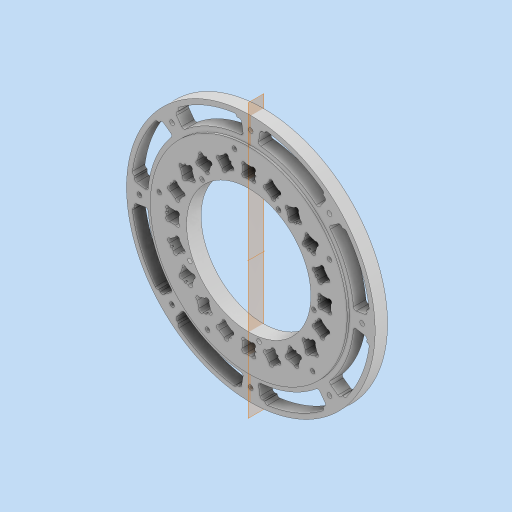
# Autodesk Inventor part: Ring_1
Saved by Autodesk Inventor 2024.2 (Build 282272000, 272)
## iProperties
Created: 2025-04-23
Part Number: Ring_1
Material: Generic
Document SubType Name: Modeling
Designer: 23661194
Density: 1 g/cm^3
Appearance: Default
Author: 23661194
Autodesk Inventor part; units mm, degrees
ref_plane "XZ Plane" through (0, 0, 0) normal (0, 1, 0) x (-1, 0, 0)
ref_plane "XY Plane" through (0, 0, 0) normal (0, 0, 1) x (1, 0, 0)
sketch "Shim Tray Slot" plane through (0, 0, 0) normal (0, 0, 1) x (1, 0, 0)
  line L0 (30.092, 109.0254) -> (29.9458, 108.3375)
  line L1 (33.5758, 105.3229) -> (31.6821, 97.1202)
  line L2 (-33.5758, 105.3229) -> (-31.6821, 97.1202)
  line L3 (-30.092, 109.0254) -> (-29.9458, 108.3375)
  arc A0 (-32.2001, 107.689) -> (-33.5758, 105.3229) centre (-31.6271, 105.7728) ccw
  arc A1 (29.1504, 95.657) -> (-29.1504, 95.657) centre (0, 0) ccw
  arc A2 (28.6337, 111.3782) -> (-28.6337, 111.3782) centre (0, 0) ccw
  arc A3 (-29.9458, 108.3375) -> (-32.2001, 107.689) centre (0, 0) ccw
  arc A4 (32.2001, 107.689) -> (29.9458, 108.3375) centre (0, 0) ccw
  arc A5 (-28.6337, 111.3782) -> (-30.092, 109.0254) centre (-28.1357, 109.4412) ccw
  arc A6 (-31.6821, 97.1202) -> (-29.1504, 95.657) centre (-29.7334, 97.5701) ccw
  arc A7 (29.1504, 95.657) -> (31.6821, 97.1202) centre (29.7309, 97.5743) ccw
  arc A8 (33.5758, 105.3229) -> (32.2001, 107.689) centre (31.6271, 105.7728) ccw
  arc A9 (30.092, 109.0254) -> (28.6337, 111.3782) centre (28.1357, 109.4412) ccw
  point P0 (0, 107.5)
  dimension "d173" = 22.5
sketch "Shim Tray Slot_1" plane through (0, 0, 0) normal (0, 0, 1) x (1, 0, 0)
  line L0 (30.092, 109.0254) -> (29.9458, 108.3375)
  line L1 (33.5758, 105.3229) -> (31.6829, 97.1237)
  line L2 (-33.5758, 105.3229) -> (-31.6821, 97.1202)
  line L3 (-30.092, 109.0254) -> (-29.9458, 108.3375)
  arc A0 (-32.2001, 107.689) -> (-33.5758, 105.3229) centre (-31.6271, 105.7728) ccw
  arc A1 (29.147, 95.658) -> (-29.1504, 95.657) centre (0, 0) ccw
  arc A2 (28.6337, 111.3782) -> (-28.6337, 111.3782) centre (0, 0) ccw
  arc A3 (-29.9458, 108.3375) -> (-32.2001, 107.689) centre (0, 0) ccw
  arc A4 (32.2001, 107.689) -> (29.9458, 108.3375) centre (0, 0) ccw
  arc A5 (-28.6337, 111.3782) -> (-30.092, 109.0254) centre (-28.1357, 109.4412) ccw
  arc A6 (-31.6821, 97.1202) -> (-29.1504, 95.657) centre (-29.7334, 97.5701) ccw
  arc A7 (29.147, 95.658) -> (31.6829, 97.1237) centre (29.7309, 97.5743) ccw
  arc A8 (33.5758, 105.3229) -> (32.2001, 107.689) centre (31.6271, 105.7728) ccw
  arc A9 (30.092, 109.0254) -> (28.6337, 111.3782) centre (28.1357, 109.4412) ccw
  line L4 (0, 0) -> (0, 107.5)
  arc A10 (33.9656, 105.2329) -> (32.3146, 108.0722) centre (31.6271, 105.7728) ccw
  line L5 (33.9656, 105.2329) -> (32.0726, 97.0337)
  arc A11 (29.0304, 95.2754) -> (32.0726, 97.0337) centre (29.7309, 97.5743) ccw
  arc A12 (29.0304, 95.2754) -> (-29.0338, 95.2743) centre (0, 0) ccw
  arc A13 (-32.0718, 97.0302) -> (-29.0338, 95.2743) centre (-29.7334, 97.5701) ccw
  line L6 (-32.0718, 97.0302) -> (-33.9656, 105.2329)
  arc A14 (-32.3146, 108.0722) -> (-33.9656, 105.2329) centre (-31.6271, 105.7728) ccw
  arc A15 (-30.4152, 108.6221) -> (-32.3146, 108.0722) centre (0, 0) ccw
  line L7 (-30.4152, 108.6221) -> (-30.4833, 108.9422)
  arc A16 (-28.7333, 111.7656) -> (-30.4833, 108.9422) centre (-28.1357, 109.4412) ccw
  arc A17 (28.7333, 111.7656) -> (-28.7333, 111.7656) centre (0, 0) ccw
  arc A18 (30.4833, 108.9422) -> (28.7333, 111.7656) centre (28.1357, 109.4412) ccw
  line L8 (30.4833, 108.9422) -> (30.4152, 108.6221)
  arc A19 (32.3146, 108.0722) -> (30.4152, 108.6221) centre (0, 0) ccw
  dimension "d182" = 0.4
  measures "d182" radial gap between concentric circles of A2 A17
sketch "Sketch1" plane through (0, 0, 0) normal (0, 0, 1) x (1, 0, 0)
  circle A0 centre (0, 0) radius 60
  circle A1 centre (0, 0) radius 120
  circle A2 centre (0, 0) radius 95
  dimension "d0" = 120
  dimension "d1" = 240
  dimension "d2" = 190
  constraints: 3 centre point, 3 coincident
  measures "d0" diameter of A0
  measures "d1" diameter of A1
  measures "d2" diameter of A2
extrude "Extrusion1" add sketch "Sketch1" along normal blind 12 contours A1 | A2
extrude "Extrusion2" add sketch "Sketch1" along normal blind 14 contours A2
sketch "Sketch2" plane through (0, 0, 14) normal (0, 0, 1) x (1, 0, 0)
  circle A0 centre (0, 0) radius 73.485
  line L0 (73.485, 0) -> (0, 0)
  line L1 (69.8884, 22.7081) -> (0, 0)
  line L2 (59.4506, 43.1934) -> (0, 0)
  line L3 (43.1934, 59.4506) -> (0, 0)
  line L4 (22.7081, 69.8884) -> (0, 0)
  line L5 (0, 73.485) -> (0, 0)
  line L6 (-22.7081, 69.8884) -> (0, 0)
  line L7 (-43.1934, 59.4506) -> (0, 0)
  line L8 (-59.4506, 43.1934) -> (0, 0)
  line L9 (-69.8884, 22.7081) -> (0, 0)
  line L10 (-73.485, 0) -> (0, 0)
  line L11 (-69.8884, -22.7081) -> (0, 0)
  line L12 (-59.4506, -43.1934) -> (0, 0)
  line L13 (-43.1934, -59.4506) -> (0, 0)
  line L14 (-22.7081, -69.8884) -> (0, 0)
  line L15 (0, -73.485) -> (0, 0)
  line L16 (22.7081, -69.8884) -> (0, 0)
  line L17 (43.1934, -59.4506) -> (0, 0)
  line L18 (59.4506, -43.1934) -> (0, 0)
  line L19 (69.8884, -22.7081) -> (0, 0)
  line L20 (-168, 0) -> (168, 0) projected
  line L21 (79.425, 5.94) -> (67.545, 5.94)
  line L22 (67.545, 5.94) -> (67.545, -5.94)
  line L23 (67.545, -5.94) -> (79.425, -5.94)
  line L24 (79.425, -5.94) -> (79.425, 5.94)
  line L25 (79.425, 5.94) -> (67.545, -5.94) construction
  line L26 (67.545, 5.94) -> (79.425, -5.94) construction
  circle A1 centre (73.485, 0) radius 2
  circle A2 centre (68.958, -4.527) radius 2.1
  circle A3 centre (78.012, -4.527) radius 2.1
  circle A4 centre (78.012, 4.527) radius 2.1
  circle A5 centre (68.958, 4.527) radius 2.1
  circle A6 centre (67.185, 0) radius 0.75
  line L27 (67.185, 0) -> (73.485, 0)
  line L28 (71.2025, 31.0051) -> (61.5914, 24.0222)
  line L29 (61.5914, 24.0222) -> (68.5743, 14.4111)
  line L30 (68.5743, 14.4111) -> (78.1854, 21.394)
  line L31 (78.1854, 21.394) -> (71.2025, 31.0051)
  line L32 (71.2025, 31.0051) -> (68.5743, 14.4111) construction
  line L33 (61.5914, 24.0222) -> (78.1854, 21.394) construction
  circle A7 centre (69.8884, 22.7081) radius 2
  circle A8 centre (68.8869, 16.3848) radius 2.1
  circle A9 centre (76.2117, 21.7066) radius 2.1
  circle A10 centre (70.8899, 29.0314) radius 2.1
  circle A11 centre (63.5651, 23.7096) radius 2.1
  circle A12 centre (64.7916, 19.0051) radius 0.75
  line L34 (64.7916, 19.0051) -> (69.8884, 22.7081)
  line L35 (55.6369, 50.6782) -> (51.9658, 39.3797)
  line L36 (51.9658, 39.3797) -> (63.2643, 35.7086)
  line L37 (63.2643, 35.7086) -> (66.9355, 47.0071)
  line L38 (66.9355, 47.0071) -> (55.6369, 50.6782)
  line L39 (55.6369, 50.6782) -> (63.2643, 35.7086) construction
  line L40 (51.9658, 39.3797) -> (66.9355, 47.0071) construction
  circle A13 centre (59.4506, 43.1934) radius 2
  circle A14 centre (62.3571, 37.489) radius 2.1
  circle A15 centre (65.155, 46.0999) radius 2.1
  circle A16 centre (56.5441, 48.8978) radius 2.1
  circle A17 centre (53.7463, 40.2869) radius 2.1
  circle A18 centre (57.5038, 37.2017) radius 0.75
  line L41 (57.5038, 37.2017) -> (59.4506, 43.1934)
  line L42 (35.7086, 63.2643) -> (39.3797, 51.9658)
  line L43 (39.3797, 51.9658) -> (50.6782, 55.6369)
  line L44 (50.6782, 55.6369) -> (47.0071, 66.9355)
  line L45 (47.0071, 66.9355) -> (35.7086, 63.2643)
  line L46 (35.7086, 63.2643) -> (50.6782, 55.6369) construction
  line L47 (39.3797, 51.9658) -> (47.0071, 66.9355) construction
  circle A19 centre (43.1934, 59.4506) radius 2
  circle A20 centre (48.8978, 56.5441) radius 2.1
  circle A21 centre (46.0999, 65.155) radius 2.1
  circle A22 centre (37.489, 62.3571) radius 2.1
  circle A23 centre (40.2869, 53.7463) radius 2.1
  circle A24 centre (45.1402, 53.459) radius 0.75
  line L48 (45.1402, 53.459) -> (43.1934, 59.4506)
  line L49 (14.4111, 68.5743) -> (24.0222, 61.5914)
  line L50 (24.0222, 61.5914) -> (31.0051, 71.2025)
  line L51 (31.0051, 71.2025) -> (21.394, 78.1854)
  line L52 (21.394, 78.1854) -> (14.4111, 68.5743)
  line L53 (14.4111, 68.5743) -> (31.0051, 71.2025) construction
  line L54 (24.0222, 61.5914) -> (21.394, 78.1854) construction
  circle A25 centre (22.7081, 69.8884) radius 2
  circle A26 centre (29.0314, 70.8899) radius 2.1
  circle A27 centre (21.7066, 76.2117) radius 2.1
  circle A28 centre (16.3848, 68.8869) radius 2.1
  circle A29 centre (23.7096, 63.5651) radius 2.1
  circle A30 centre (27.8049, 66.1853) radius 0.75
  line L55 (27.8049, 66.1853) -> (22.7081, 69.8884)
  line L56 (-5.94, 67.545) -> (5.94, 67.545)
  line L57 (5.94, 67.545) -> (5.94, 79.425)
  line L58 (5.94, 79.425) -> (-5.94, 79.425)
  line L59 (-5.94, 79.425) -> (-5.94, 67.545)
  line L60 (-5.94, 67.545) -> (5.94, 79.425) construction
  line L61 (5.94, 67.545) -> (-5.94, 79.425) construction
  circle A31 centre (0, 73.485) radius 2
  circle A32 centre (4.527, 78.012) radius 2.1
  circle A33 centre (-4.527, 78.012) radius 2.1
  circle A34 centre (-4.527, 68.958) radius 2.1
  circle A35 centre (4.527, 68.958) radius 2.1
  circle A36 centre (6.3, 73.485) radius 0.75
  line L62 (6.3, 73.485) -> (0, 73.485)
  line L63 (-24.0222, 61.5914) -> (-14.4111, 68.5743)
  line L64 (-14.4111, 68.5743) -> (-21.394, 78.1854)
  line L65 (-21.394, 78.1854) -> (-31.0051, 71.2025)
  line L66 (-31.0051, 71.2025) -> (-24.0222, 61.5914)
  line L67 (-24.0222, 61.5914) -> (-21.394, 78.1854) construction
  line L68 (-14.4111, 68.5743) -> (-31.0051, 71.2025) construction
  circle A37 centre (-22.7081, 69.8884) radius 2
  circle A38 centre (-21.7066, 76.2117) radius 2.1
  circle A39 centre (-29.0314, 70.8899) radius 2.1
  circle A40 centre (-23.7096, 63.5651) radius 2.1
  circle A41 centre (-16.3848, 68.8869) radius 2.1
  circle A42 centre (-17.6113, 73.5914) radius 0.75
  line L69 (-17.6113, 73.5914) -> (-22.7081, 69.8884)
  line L70 (-39.3797, 51.9658) -> (-35.7086, 63.2643)
  line L71 (-35.7086, 63.2643) -> (-47.0071, 66.9355)
  line L72 (-47.0071, 66.9355) -> (-50.6782, 55.6369)
  line L73 (-50.6782, 55.6369) -> (-39.3797, 51.9658)
  line L74 (-39.3797, 51.9658) -> (-47.0071, 66.9355) construction
  line L75 (-35.7086, 63.2643) -> (-50.6782, 55.6369) construction
  circle A43 centre (-43.1934, 59.4506) radius 2
  circle A44 centre (-46.0999, 65.155) radius 2.1
  circle A45 centre (-48.8978, 56.5441) radius 2.1
  circle A46 centre (-40.2869, 53.7463) radius 2.1
  circle A47 centre (-37.489, 62.3571) radius 2.1
  circle A48 centre (-41.2466, 65.4423) radius 0.75
  line L76 (-41.2466, 65.4423) -> (-43.1934, 59.4506)
  line L77 (-51.9658, 39.3797) -> (-55.6369, 50.6782)
  line L78 (-55.6369, 50.6782) -> (-66.9355, 47.0071)
  line L79 (-66.9355, 47.0071) -> (-63.2643, 35.7086)
  line L80 (-63.2643, 35.7086) -> (-51.9658, 39.3797)
  line L81 (-51.9658, 39.3797) -> (-66.9355, 47.0071) construction
  line L82 (-55.6369, 50.6782) -> (-63.2643, 35.7086) construction
  circle A49 centre (-59.4506, 43.1934) radius 2
  circle A50 centre (-65.155, 46.0999) radius 2.1
  circle A51 centre (-62.3571, 37.489) radius 2.1
  circle A52 centre (-53.7463, 40.2869) radius 2.1
  circle A53 centre (-56.5441, 48.8978) radius 2.1
  circle A54 centre (-61.3974, 49.1851) radius 0.75
  line L83 (-61.3974, 49.1851) -> (-59.4506, 43.1934)
  line L84 (-61.5914, 24.0222) -> (-71.2025, 31.0051)
  line L85 (-71.2025, 31.0051) -> (-78.1854, 21.394)
  line L86 (-78.1854, 21.394) -> (-68.5743, 14.4111)
  line L87 (-68.5743, 14.4111) -> (-61.5914, 24.0222)
  line L88 (-61.5914, 24.0222) -> (-78.1854, 21.394) construction
  line L89 (-71.2025, 31.0051) -> (-68.5743, 14.4111) construction
  circle A55 centre (-69.8884, 22.7081) radius 2
  circle A56 centre (-76.2117, 21.7066) radius 2.1
  circle A57 centre (-68.8869, 16.3848) radius 2.1
  circle A58 centre (-63.5651, 23.7096) radius 2.1
  circle A59 centre (-70.8899, 29.0314) radius 2.1
  circle A60 centre (-74.9852, 26.4112) radius 0.75
  line L90 (-74.9852, 26.4112) -> (-69.8884, 22.7081)
  line L91 (-67.545, 5.94) -> (-79.425, 5.94)
  line L92 (-79.425, 5.94) -> (-79.425, -5.94)
  line L93 (-79.425, -5.94) -> (-67.545, -5.94)
  line L94 (-67.545, -5.94) -> (-67.545, 5.94)
  line L95 (-67.545, 5.94) -> (-79.425, -5.94) construction
  line L96 (-79.425, 5.94) -> (-67.545, -5.94) construction
  circle A61 centre (-73.485, 0) radius 2
  circle A62 centre (-78.012, -4.527) radius 2.1
  circle A63 centre (-68.958, -4.527) radius 2.1
  circle A64 centre (-68.958, 4.527) radius 2.1
  circle A65 centre (-78.012, 4.527) radius 2.1
  circle A66 centre (-79.785, 0) radius 0.75
  line L97 (-79.785, 0) -> (-73.485, 0)
  line L98 (-68.5743, -14.4111) -> (-78.1854, -21.394)
  line L99 (-78.1854, -21.394) -> (-71.2025, -31.0051)
  line L100 (-71.2025, -31.0051) -> (-61.5914, -24.0222)
  line L101 (-61.5914, -24.0222) -> (-68.5743, -14.4111)
  line L102 (-68.5743, -14.4111) -> (-71.2025, -31.0051) construction
  line L103 (-78.1854, -21.394) -> (-61.5914, -24.0222) construction
  circle A67 centre (-69.8884, -22.7081) radius 2
  circle A68 centre (-70.8899, -29.0314) radius 2.1
  circle A69 centre (-63.5651, -23.7096) radius 2.1
  circle A70 centre (-68.8869, -16.3848) radius 2.1
  circle A71 centre (-76.2117, -21.7066) radius 2.1
  circle A72 centre (-74.9852, -26.4112) radius 0.75
  line L104 (-74.9852, -26.4112) -> (-69.8884, -22.7081)
  line L105 (-63.2643, -35.7086) -> (-66.9355, -47.0071)
  line L106 (-66.9355, -47.0071) -> (-55.6369, -50.6782)
  line L107 (-55.6369, -50.6782) -> (-51.9658, -39.3797)
  line L108 (-51.9658, -39.3797) -> (-63.2643, -35.7086)
  line L109 (-63.2643, -35.7086) -> (-55.6369, -50.6782) construction
  line L110 (-66.9355, -47.0071) -> (-51.9658, -39.3797) construction
  circle A73 centre (-59.4506, -43.1934) radius 2
  circle A74 centre (-56.5441, -48.8978) radius 2.1
  circle A75 centre (-53.7463, -40.2869) radius 2.1
  circle A76 centre (-62.3571, -37.489) radius 2.1
  circle A77 centre (-65.155, -46.0999) radius 2.1
  circle A78 centre (-61.3974, -49.1851) radius 0.75
  line L111 (-61.3974, -49.1851) -> (-59.4506, -43.1934)
  line L112 (-50.6782, -55.6369) -> (-47.0071, -66.9355)
  line L113 (-47.0071, -66.9355) -> (-35.7086, -63.2643)
  line L114 (-35.7086, -63.2643) -> (-39.3797, -51.9658)
  line L115 (-39.3797, -51.9658) -> (-50.6782, -55.6369)
  line L116 (-50.6782, -55.6369) -> (-35.7086, -63.2643) construction
  line L117 (-47.0071, -66.9355) -> (-39.3797, -51.9658) construction
  circle A79 centre (-43.1934, -59.4506) radius 2
  circle A80 centre (-37.489, -62.3571) radius 2.1
  circle A81 centre (-40.2869, -53.7463) radius 2.1
  circle A82 centre (-48.8978, -56.5441) radius 2.1
  circle A83 centre (-46.0999, -65.155) radius 2.1
  circle A84 centre (-41.2466, -65.4423) radius 0.75
  line L118 (-41.2466, -65.4423) -> (-43.1934, -59.4506)
  line L119 (-31.0051, -71.2025) -> (-21.394, -78.1854)
  line L120 (-21.394, -78.1854) -> (-14.4111, -68.5743)
  line L121 (-14.4111, -68.5743) -> (-24.0222, -61.5914)
  line L122 (-24.0222, -61.5914) -> (-31.0051, -71.2025)
  line L123 (-31.0051, -71.2025) -> (-14.4111, -68.5743) construction
  line L124 (-21.394, -78.1854) -> (-24.0222, -61.5914) construction
  circle A85 centre (-22.7081, -69.8884) radius 2
  circle A86 centre (-16.3848, -68.8869) radius 2.1
  circle A87 centre (-23.7096, -63.5651) radius 2.1
  circle A88 centre (-29.0314, -70.8899) radius 2.1
  circle A89 centre (-21.7066, -76.2117) radius 2.1
  circle A90 centre (-17.6113, -73.5914) radius 0.75
  line L125 (-17.6113, -73.5914) -> (-22.7081, -69.8884)
  line L126 (-5.94, -79.425) -> (5.94, -79.425)
  line L127 (5.94, -79.425) -> (5.94, -67.545)
  line L128 (5.94, -67.545) -> (-5.94, -67.545)
  line L129 (-5.94, -67.545) -> (-5.94, -79.425)
  line L130 (-5.94, -79.425) -> (5.94, -67.545) construction
  line L131 (5.94, -79.425) -> (-5.94, -67.545) construction
  circle A91 centre (0, -73.485) radius 2
  circle A92 centre (4.527, -68.958) radius 2.1
  circle A93 centre (-4.527, -68.958) radius 2.1
  circle A94 centre (-4.527, -78.012) radius 2.1
  circle A95 centre (4.527, -78.012) radius 2.1
  circle A96 centre (6.3, -73.485) radius 0.75
  line L132 (6.3, -73.485) -> (0, -73.485)
  line L133 (21.394, -78.1854) -> (31.0051, -71.2025)
  line L134 (31.0051, -71.2025) -> (24.0222, -61.5914)
  line L135 (24.0222, -61.5914) -> (14.4111, -68.5743)
  line L136 (14.4111, -68.5743) -> (21.394, -78.1854)
  line L137 (21.394, -78.1854) -> (24.0222, -61.5914) construction
  line L138 (31.0051, -71.2025) -> (14.4111, -68.5743) construction
  circle A97 centre (22.7081, -69.8884) radius 2
  circle A98 centre (23.7096, -63.5651) radius 2.1
  circle A99 centre (16.3848, -68.8869) radius 2.1
  circle A100 centre (21.7066, -76.2117) radius 2.1
  circle A101 centre (29.0314, -70.8899) radius 2.1
  circle A102 centre (27.8049, -66.1853) radius 0.75
  line L139 (27.8049, -66.1853) -> (22.7081, -69.8884)
  line L140 (78.1854, -21.394) -> (68.5743, -14.4111)
  line L141 (68.5743, -14.4111) -> (61.5914, -24.0222)
  line L142 (61.5914, -24.0222) -> (71.2025, -31.0051)
  line L143 (71.2025, -31.0051) -> (78.1854, -21.394)
  line L144 (78.1854, -21.394) -> (61.5914, -24.0222) construction
  line L145 (68.5743, -14.4111) -> (71.2025, -31.0051) construction
  circle A103 centre (69.8884, -22.7081) radius 2
  circle A104 centre (63.5651, -23.7096) radius 2.1
  circle A105 centre (70.8899, -29.0314) radius 2.1
  circle A106 centre (76.2117, -21.7066) radius 2.1
  circle A107 centre (68.8869, -16.3848) radius 2.1
  circle A108 centre (64.7916, -19.0051) radius 0.75
  line L146 (64.7916, -19.0051) -> (69.8884, -22.7081)
  line L147 (47.0071, -66.9355) -> (50.6782, -55.6369)
  line L148 (50.6782, -55.6369) -> (39.3797, -51.9658)
  line L149 (39.3797, -51.9658) -> (35.7086, -63.2643)
  line L150 (35.7086, -63.2643) -> (47.0071, -66.9355)
  line L151 (47.0071, -66.9355) -> (39.3797, -51.9658) construction
  line L152 (50.6782, -55.6369) -> (35.7086, -63.2643) construction
  circle A109 centre (43.1934, -59.4506) radius 2
  circle A110 centre (40.2869, -53.7463) radius 2.1
  circle A111 centre (37.489, -62.3571) radius 2.1
  circle A112 centre (46.0999, -65.155) radius 2.1
  circle A113 centre (48.8978, -56.5441) radius 2.1
  circle A114 centre (45.1402, -53.459) radius 0.75
  line L153 (45.1402, -53.459) -> (43.1934, -59.4506)
  line L154 (66.9355, -47.0071) -> (63.2643, -35.7086)
  line L155 (63.2643, -35.7086) -> (51.9658, -39.3797)
  line L156 (51.9658, -39.3797) -> (55.6369, -50.6782)
  line L157 (55.6369, -50.6782) -> (66.9355, -47.0071)
  line L158 (66.9355, -47.0071) -> (51.9658, -39.3797) construction
  line L159 (63.2643, -35.7086) -> (55.6369, -50.6782) construction
  circle A115 centre (59.4506, -43.1934) radius 2
  circle A116 centre (53.7463, -40.2869) radius 2.1
  circle A117 centre (56.5441, -48.8978) radius 2.1
  circle A118 centre (65.155, -46.0999) radius 2.1
  circle A119 centre (62.3571, -37.489) radius 2.1
  circle A120 centre (57.5038, -37.2017) radius 0.75
  line L160 (57.5038, -37.2017) -> (59.4506, -43.1934)
  point P0 (68.8025, -29.2614)
  point P1 (72.9462, -28.6052)
  point P2 (76.4417, -23.794)
  point P3 (75.7854, -19.6503)
  point P4 (70.9742, -16.1548)
  point P5 (66.8306, -16.8111)
  point P6 (63.3351, -21.6223)
  point P7 (63.9913, -25.7659)
  point P8 (52.8825, -42.201)
  point P9 (54.7202, -47.8569)
  point P10 (58.4582, -49.7615)
  point P11 (64.1141, -47.9238)
  point P12 (66.0187, -44.1858)
  point P13 (64.181, -38.5299)
  point P14 (60.443, -36.6253)
  point P15 (54.7871, -38.463)
  point P16 (36.6253, -60.443)
  point P17 (38.5299, -64.181)
  point P18 (44.1858, -66.0187)
  point P19 (47.9238, -64.1141)
  point P20 (49.7615, -58.4582)
  point P21 (47.8569, -54.7202)
  point P22 (42.201, -52.8825)
  point P23 (38.463, -54.7871)
  point P24 (19.6503, -75.7854)
  point P25 (23.794, -76.4417)
  point P26 (28.6052, -72.9462)
  point P27 (29.2614, -68.8025)
  point P28 (25.7659, -63.9913)
  point P29 (21.6223, -63.3351)
  point P30 (16.8111, -66.8306)
  point P31 (16.1548, -70.9742)
  point P32 (5.94, -70.5115)
  point P33 (2.9735, -67.545)
  point P34 (-2.9735, -67.545)
  point P35 (-5.94, -70.5115)
  point P36 (-5.94, -76.4585)
  point P37 (-2.9735, -79.425)
  point P38 (2.9735, -79.425)
  point P39 (5.94, -76.4585)
  point P40 (-21.6223, -63.3351)
  point P41 (-25.7659, -63.9913)
  point P42 (-29.2614, -68.8025)
  point P43 (-28.6052, -72.9462)
  point P44 (-23.794, -76.4417)
  point P45 (-19.6503, -75.7854)
  point P46 (-16.1548, -70.9742)
  point P47 (-16.8111, -66.8306)
  point P48 (-49.7615, -58.4582)
  point P49 (-47.9238, -64.1141)
  point P50 (-44.1858, -66.0187)
  point P51 (-38.5299, -64.181)
  point P52 (-36.6253, -60.443)
  point P53 (-38.463, -54.7871)
  point P54 (-42.201, -52.8825)
  point P55 (-47.8569, -54.7202)
  point P56 (-54.7202, -47.8569)
  point P57 (-52.8825, -42.201)
  point P58 (-54.7871, -38.463)
  point P59 (-60.443, -36.6253)
  point P60 (-64.181, -38.5299)
  point P61 (-66.0187, -44.1858)
  point P62 (-64.1141, -47.9238)
  point P63 (-58.4582, -49.7615)
  point P64 (-66.8306, -16.8111)
  point P65 (-70.9742, -16.1548)
  point P66 (-75.7854, -19.6503)
  point P67 (-76.4417, -23.794)
  point P68 (-72.9462, -28.6052)
  point P69 (-68.8025, -29.2614)
  point P70 (-63.9913, -25.7659)
  point P71 (-63.3351, -21.6223)
  point P72 (-67.545, 2.9735)
  point P73 (-70.5115, 5.94)
  point P74 (-76.4585, 5.94)
  point P75 (-79.425, 2.9735)
  point P76 (-79.425, -2.9735)
  point P77 (-76.4585, -5.94)
  point P78 (-70.5115, -5.94)
  point P79 (-67.545, -2.9735)
  point P80 (-63.3351, 21.6223)
  point P81 (-63.9913, 25.7659)
  point P82 (-68.8025, 29.2614)
  point P83 (-72.9462, 28.6052)
  point P84 (-76.4417, 23.794)
  point P85 (-75.7854, 19.6503)
  point P86 (-70.9742, 16.1548)
  point P87 (-66.8306, 16.8111)
  point P88 (-54.7871, 38.463)
  point P89 (-52.8825, 42.201)
  point P90 (-54.7202, 47.8569)
  point P91 (-58.4582, 49.7615)
  point P92 (-64.1141, 47.9238)
  point P93 (-66.0187, 44.1858)
  point P94 (-64.181, 38.5299)
  point P95 (-60.443, 36.6253)
  point P96 (-42.201, 52.8825)
  point P97 (-38.463, 54.7871)
  point P98 (-36.6253, 60.443)
  point P99 (-38.5299, 64.181)
  point P100 (-44.1858, 66.0187)
  point P101 (-47.9238, 64.1141)
  point P102 (-49.7615, 58.4582)
  point P103 (-47.8569, 54.7202)
  point P104 (-16.8111, 66.8306)
  point P105 (-16.1548, 70.9742)
  point P106 (-19.6503, 75.7854)
  point P107 (-23.794, 76.4417)
  point P108 (-28.6052, 72.9462)
  point P109 (-29.2614, 68.8025)
  point P110 (-25.7659, 63.9913)
  point P111 (-21.6223, 63.3351)
  point P112 (-5.94, 70.5115)
  point P113 (-2.9735, 67.545)
  point P114 (2.9735, 67.545)
  point P115 (5.94, 70.5115)
  point P116 (5.94, 76.4585)
  point P117 (2.9735, 79.425)
  point P118 (-2.9735, 79.425)
  point P119 (-5.94, 76.4585)
  point P120 (16.1548, 70.9742)
  point P121 (16.8111, 66.8306)
  point P122 (21.6223, 63.3351)
  point P123 (25.7659, 63.9913)
  point P124 (29.2614, 68.8025)
  point P125 (28.6052, 72.9462)
  point P126 (23.794, 76.4417)
  point P127 (19.6503, 75.7854)
  point P128 (36.6253, 60.443)
  point P129 (38.463, 54.7871)
  point P130 (42.201, 52.8825)
  point P131 (47.8569, 54.7202)
  point P132 (49.7615, 58.4582)
  point P133 (47.9238, 64.1141)
  point P134 (44.1858, 66.0187)
  point P135 (38.5299, 64.181)
  point P136 (64.181, 38.5299)
  point P137 (66.0187, 44.1858)
  point P138 (64.1141, 47.9238)
  point P139 (58.4582, 49.7615)
  point P140 (54.7202, 47.8569)
  point P141 (52.8825, 42.201)
  point P142 (54.7871, 38.463)
  point P143 (60.443, 36.6253)
  point P144 (63.9913, 25.7659)
  point P145 (63.3351, 21.6223)
  point P146 (66.8306, 16.8111)
  point P147 (70.9742, 16.1548)
  point P148 (75.7854, 19.6503)
  point P149 (76.4417, 23.794)
  point P150 (72.9462, 28.6052)
  point P151 (68.8025, 29.2614)
  point P152 (70.5115, 5.94)
  point P153 (67.545, 2.9735)
  point P154 (67.545, -2.9735)
  point P155 (70.5115, -5.94)
  point P156 (76.4585, -5.94)
  point P157 (79.425, -2.9735)
  point P158 (79.425, 2.9735)
  point P159 (76.4585, 5.94)
  dimension "d7" = 146.97
  dimension "d123" = -36
  dimension "d124" = -72
  dimension "d125" = -108
  dimension "d126" = -144
  dimension "d127" = -180
  dimension "d128" = -216
  dimension "d129" = -252
  dimension "d130" = -288
  dimension "d131" = -324
  dimension "d132" = 0
  dimension "d133" = -36
  dimension "d134" = -72
  dimension "d135" = -108
  dimension "d136" = -144
  dimension "d137" = 180
  dimension "d138" = -216
  dimension "d139" = -252
  dimension "d140" = -288
  dimension "d141" = -324
  dimension "d120" = 360
  dimension "d122" = 0
  constraints: 40 end point, 2 horizontal, 1 coincident, 1 horizontal alignment, 84 other
  measures "d122" vertical extent of L0
extrude "Extrusion3" cut sketch "Sketch2" against normal blind 12 contours L0 A1 A0 | L20 A1 A0 | A0 A1 L0 | A0 A1 L20 | A1 L0 A6 L22 A5 L21 A0 | A0 L21 A4 L24 L20 A1 | A1 L20 L24 A3 L23 A0 | A0 L23 A2 L22 A6 L0 A1 | A6 L22 L0 | L0 L22 A6 | L30 A8 L29 A12 L34 A7 A0 | A0 A7 L28 A10 L31 A9 L30 | A4 L24 L21 | L21 L24 A4 | A5 L22 L21 | L21 L22 A5 | L140 A106 L143 A105 L142 A0 A103 | A0 A103 L146 A108 L141 A107 L140 | A2 L22 L23 | L23 L22 A2 | A3 L24 L23 | L23 L24 A3 | A7 L34 A0 | A0 A7 | A8 L29 L30 | L30 L29 A8 | A9 L31 L30 | L30 L31 A9 | A103 A0 | A0 L146 A103 | A106 L143 L140 | L140 L143 A106 | A107 L141 L140 | L140 L141 A107 | L1 A7 A0 | L34 A7 L1 | L34 A12 L29 L1 A7 | A0 A103 L19 | L19 A103 L146 | A103 L19 L141 A108 L146 | A7 L1 L29 A11 L28 A0 | L34 L29 A12 | A12 L29 L34 | A10 L28 L31 | L31 L28 A10 | A0 L142 A104 L141 L19 A103 | L146 L141 A108 | A108 L141 L146 | A105 L142 L143 | L143 L142 A105 | A17 L35 L36 L2 | L2 L36 A17 | A23 L42 L3 | L3 L42 L43 A23 | L49 A28 L52 A0 A25 L4 | L4 A25 L55 A30 L50 A29 L49 | L56 A34 L59 A0 A31 L5 | L5 A31 A0 A36 L57 A35 L56 | L63 A40 L66 A0 A37 L6 | L6 A37 A0 L64 A41 L63 | A46 L73 L70 L7 | L7 L70 A46 | A52 L80 L8 | L8 L80 L77 A52 | L87 A57 L86 A0 A55 L9 | L9 A55 A0 L84 A58 L87 | L94 A63 L93 A0 A61 L10 | L10 A61 A0 L91 A64 L94 | L101 A69 L100 A0 A67 L11 | L11 A67 A0 L98 A70 L101 | A75 L107 L108 L12 | L12 L108 A75 | A81 L114 L13 | L13 L114 L115 A81 | L121 A86 L120 A0 A85 L14 | L14 A85 A0 L122 A87 L121 | L128 A92 L127 A96 A0 A91 L15 | L15 A91 A0 L129 A93 L128 | L135 A98 L134 A102 L139 A97 L16 | L16 A97 A0 L136 A99 L135 | A110 L148 L149 L17 | L17 L149 A110 | A116 L155 L18 | L18 L155 L156 A116 | A11 L28 L29 | L29 L28 A11 | L36 L35 A17 L2 | L2 A17 L36 | L35 A16 A0 A13 L2 A17 | A17 L2 A13 L41 A18 L36 | L42 A23 L3 | L3 A23 L43 L42 | L42 A22 A0 A19 L3 A23 | A23 L3 A19 L48 A24 L43 | A25 A0 L4 | L4 L55 A25 | A28 L52 L49 | L49 L52 A28 | A29 L50 L49 | L49 L50 A29 | A31 A0 L5 | L5 A0 A31 | A34 L59 L56 | L56 L59 A34 | A35 L57 L56 | L56 L57 A35 | A37 A0 L6 | L6 A0 A37 | A40 L66 L63 | L63 L66 A40 | A41 L64 L63 | L63 L64 A41 | L70 L73 A46 L7 | L7 A46 L70 | L73 A45 A0 A43 L7 A46 | L80 A52 L8 | L8 A52 L77 L80 | L80 A51 A0 A49 L8 A52 | A55 A0 L9 | L9 A0 A55 | A57 L86 L87 | L87 L86 A57 | A58 L84 L87 | L87 L84 A58 | A61 A0 L10 | L10 A0 A61 | A63 L93 L94 | L94 L93 A63 | A64 L91 L94 | L94 L91 A64 | A67 A0 L11 | L11 A0 A67 | A69 L100 L101 | L101 L100 A69 | A70 L98 L101 | L101 L98 A70 | L108 L107 A75 L12 | L12 A75 L108 | A75 L12 A73 A0 A76 L108 | L114 A81 L13 | L13 A81 L115 L114 | A81 L13 A79 A0 A82 L115 | A85 A0 L14 | L14 A0 A85 | A86 L120 L121 | L121 L120 A86 | A87 L122 L121 | L121 L122 A87 | A91 A0 L15 | L15 A0 A91 | A92 L127 L128 | L128 L127 A92 | A93 L129 L128 | L128 L129 A93 | A97 L139 L16 | L16 A0 A97 | A98 L134 L135 | L135 L134 A98 | A99 L136 L135 | L135 L136 A99 | L149 L148 A110 L17 | L17 A110 L149 | L148 A114 L153 A109 L17 A110 | A110 L17 A109 A0 A111 L149 | L155 A116 L18 | L18 A116 L156 L155 | L155 A120 L160 A115 L18 A116 | A116 L18 A115 A0 A117 L156 | A104 L142 L141 | L141 L142 A104 | A14 L36 L37 A0 | A0 L37 A14 | A119 L154 A0 | A0 L154 L155 A119 | A16 A0 L35 | L35 A0 A16 | A18 L41 L36 | A22 A0 L45 L42 | L42 L45 A0 A22 | A24 L48 L43 | A0 A25 | A0 A25 L55 | A0 L52 A27 L51 A26 L50 A25 | A25 A0 L50 A30 L55 | L62 A31 A0 | A0 A31 L62 | A0 L59 A33 L58 A32 L57 A36 L62 A31 | A31 L62 A36 A0 | L69 A37 A0 | A0 A37 L69 | A0 L66 A39 L65 A38 L64 A42 L69 A37 | L7 A43 A0 A47 L70 A46 | A45 A0 L73 | L73 A0 A45 | L8 A49 A0 A53 L77 A52 | A51 A0 L79 L80 | L80 L79 A0 A51 | L90 A55 A0 | A0 A55 L90 | A0 L86 A56 L85 A60 L90 A55 | L20 A61 A0 | A0 A61 L20 | A61 L20 A66 L92 A65 L91 A0 | A0 L93 A62 L92 A66 L20 A61 | L104 A67 A0 | A0 A67 L104 | A67 L104 A72 L99 A71 L98 A0 | A75 L107 A74 A0 A73 L12 | A76 A0 L105 L108 | L108 L105 A0 A76 | A81 L114 A80 A0 A79 L13 | A82 A0 L115 | L115 A0 A82 | L125 A85 A0 | A0 A85 L125 | A85 L125 A90 L120 A89 L119 A88 L122 A0 | L132 A91 A0 | A0 A91 L132 | A0 A96 L132 A91 | A91 L132 A96 L127 A95 L126 A94 L129 A0 | A0 A97 | L139 A97 A0 | L139 A102 L134 A0 A97 | A97 A0 L134 A101 L133 A100 L136 | L148 L153 A114 | A111 A0 L150 L149 | L149 L150 A0 A111 | L155 L160 A120 | A117 A0 L156 | L156 A0 A117 | L37 L36 A14 A0 | A0 A14 L37 | L36 A18 L41 A13 A0 A14 | L154 A119 A0 | A0 A119 L155 L154 | A119 A0 A115 L160 A120 L155 | A13 A0 L2 | L2 L41 A13 | L35 L38 A16 A0 | A0 A16 L38 L35 | A16 L38 A15 L37 A14 A0 A13 | L41 A18 L36 | A19 A0 L3 | L3 L48 A19 | A22 L45 A0 | A22 L45 A21 L44 A20 A0 A19 | A0 L45 A22 | L48 A24 L43 | L48 A19 A0 A20 L43 A24 | L55 L50 A30 | A30 L50 L55 | A36 L62 L57 A0 | A0 L57 A36 | A37 L69 A42 L64 A0 | A43 A0 L7 | L7 A0 A43 | A47 A0 L71 L70 | L70 L71 A0 A47 | L73 L72 A45 A0 | A0 A45 L72 L73 | A49 A0 L8 | L8 A0 A49 | A51 L79 A0 | A53 A0 L77 | L77 A0 A53 | A55 L90 A60 L85 A59 L84 A0 | A0 L100 A68 L99 A72 L104 A67 | A73 A0 L12 | L12 A0 A73 | A74 A0 L107 | L107 A0 A74 | A0 L105 A76 | A79 A0 L13 | L13 A0 A79 | A80 A0 L113 L114 | L114 L113 A0 A80 | L115 L112 A82 A0 | A0 A82 L112 L115 | A0 L120 A90 L125 A85 | A96 L127 A0 | A0 L127 L132 A96 | L139 L134 A102 | A102 L134 L139 | A109 L153 L17 | L17 A0 A109 | L148 A114 L153 | A114 L148 A113 A0 A109 L153 | A111 L150 A0 | A0 A109 A113 L147 A112 L150 A111 | A0 L150 A111 | A115 L160 L18 | L18 A0 A115 | L155 A120 L160 | L156 L157 A117 A0 | A0 A117 L157 L156 | A0 A115 A119 L154 A118 L157 A117 | A0 A13 | A0 A13 L41 | A20 L43 A0 | A0 L43 L44 A20 | A0 A19 | A0 A19 L48 | A27 L51 L52 | L52 L51 A27 | A36 L57 L62 | A33 L58 L59 | L59 L58 A33 | L69 L64 A42 | A42 L64 L69 | A0 L71 A47 | A39 L65 L66 | L66 L65 A39 | L76 A43 A0 | A0 A43 L76 | A0 A45 L72 A44 L71 A48 L76 A43 | A47 L71 A0 | A0 A43 L76 A48 L71 A47 | A0 L77 L78 A53 | L83 A49 A0 | A0 A49 L83 | A0 A51 L79 A50 L78 A54 L83 A49 | L79 A51 A0 | A0 A53 L78 L77 | A0 A49 L83 A54 L78 A53 | L90 L85 A60 | A60 L85 L90 | A56 L85 L86 | L86 L85 A56 | A59 L85 L84 | L84 L85 A59 | A66 L92 L20 | L20 L92 A66 | A65 L92 L91 | L91 L92 A65 | A62 L92 L93 | L93 L92 A62 | L104 L99 A72 | A72 L99 L104 | A71 L99 L98 | L98 L99 A71 | A68 L99 L100 | L100 L99 A68 | L111 A73 A0 | A0 A73 L111 | A73 L111 A78 L106 A77 L105 A76 A0 | L107 L106 A74 A0 | A0 A74 L106 L107 | A74 L106 A78 L111 A73 A0 | A0 A76 L105 | L118 A79 A0 | A0 A79 L118 | A79 L118 A84 L113 A83 L112 A82 A0 | A80 L113 A84 L118 A79 A0 | A0 L113 A80 | L125 L120 A90 | A90 L120 L125 | A80 L113 A0 | A88 L119 L122 | L122 L119 A88 | L132 L127 A96 | A94 L126 L129 | L129 L126 A94 | A100 L133 L136 | L136 L133 A100 | A0 A109 | L153 A109 A0 | A0 A115 | L160 A115 A0 | A113 L147 L148 A0 | A0 L148 A113 | A15 L38 L37 | L37 L38 A15 | A118 L157 L154 | L154 L157 A118 | L43 A20 A0 | A0 A20 L44 L43 | A26 L51 L50 | L50 L51 A26 | A21 L44 L45 | L45 L44 A21 | A44 L71 L72 | L72 L71 A44 | A50 L78 L79 | L79 L78 A50 | A77 L106 L105 | L105 L106 A77 | A83 L113 L112 | L112 L113 A83 | A101 L133 L134 | L134 L133 A101 | L148 A0 A113 | A112 L147 L150 | L150 L147 A112 | L148 L147 A113 A0 | A32 L58 L57 | L57 L58 A32 | A38 L65 L64 | L64 L65 A38 | A48 L76 L71 | A48 L71 L76 | A54 L83 L78 | A54 L78 L83 | L111 L106 A78 | A78 L106 L111 | L118 L113 A84 | A84 L113 L118 | A89 L119 L120 | L120 L119 A89 | A95 L126 L127 | L127 L126 A95 picked at (67.5888, -0.4081) picked at (67.5888, 0.4081) picked at (5.8996, 72.9937) picked at (5.8996, -72.9937) picked at (-79.3812, -0.4081) picked at (-79.3812, 0.4081)
extrude "Extrusion4" cut sketch "Sketch2" against normal blind 2 contours A6 L22 L0 | L0 L22 A6 | L22 A6 L0 | L0 A6 L22 | L34 L29 A12 | A12 L29 L34 | A12 L29 | L146 L141 A108 | A108 L141 L146 | L141 A108 | A18 L41 L36 | L36 A18 | A24 L48 L43 | L43 A24 | A114 L148 | L148 L153 A114 | A120 L155 | L155 L160 A120 | L41 A18 L36 | L48 A24 L43 | L55 L50 A30 | A30 L50 L55 | L50 A30 | A36 L62 L57 A0 | A0 L57 A36 | L57 A0 A36 | A96 L127 A0 | A0 L127 L132 A96 | A96 A0 L127 | L139 L134 A102 | A102 L134 L139 | A102 L134 | L148 A114 L153 | L155 A120 L160 | A0 L57 A36 | A36 L57 L62 | L69 L64 A42 | A42 L64 L69 | L64 A42 | L90 L85 A60 | A60 L85 L90 | A66 L92 L20 | L20 L92 A66 | L104 L99 A72 | A72 L99 L104 | L125 L120 A90 | A90 L120 L125 | A90 L120 | L132 L127 A96 | A0 A96 L127 | A60 L85 | L92 A66 L20 | L20 A66 L92 | L99 A72 | A48 L76 L71 | L71 A48 | A48 L71 L76 | A54 L83 L78 | L78 A54 | A54 L78 L83 | L111 L106 A78 | A78 L106 L111 | A78 L106 | L118 L113 A84 | A84 L113 L118 | A84 L113
extrude "Extrusion5" cut sketch "Sketch2" against normal through all contours L0 A1 A0 | L20 A1 A0 | A0 A1 L0 | A0 A1 L20 | A7 L34 A0 | A0 A7 | A103 A0 | A0 L146 A103 | L1 A7 A0 | L34 A7 L1 | A0 A103 L19 | L19 A103 L146 | A25 A0 L4 | L4 L55 A25 | A31 A0 L5 | L5 A0 A31 | A37 A0 L6 | L6 A0 A37 | A55 A0 L9 | L9 A0 A55 | A61 A0 L10 | L10 A0 A61 | A67 A0 L11 | L11 A0 A67 | A85 A0 L14 | L14 A0 A85 | A91 A0 L15 | L15 A0 A91 | A97 L139 L16 | L16 A0 A97 | A0 A25 | A0 A25 L55 | L62 A31 A0 | A0 A31 L62 | L69 A37 A0 | A0 A37 L69 | L90 A55 A0 | A0 A55 L90 | L20 A61 A0 | A0 A61 L20 | L104 A67 A0 | A0 A67 L104 | L125 A85 A0 | A0 A85 L125 | L132 A91 A0 | A0 A91 L132 | A0 A97 | L139 A97 A0 | A13 A0 L2 | L2 L41 A13 | A19 A0 L3 | L3 L48 A19 | A43 A0 L7 | L7 A0 A43 | A49 A0 L8 | L8 A0 A49 | A73 A0 L12 | L12 A0 A73 | A79 A0 L13 | L13 A0 A79 | A109 L153 L17 | L17 A0 A109 | A115 L160 L18 | L18 A0 A115 | A0 A13 | A0 A13 L41 | A0 A19 | A0 A19 L48 | L76 A43 A0 | A0 A43 L76 | L83 A49 A0 | A0 A49 L83 | L111 A73 A0 | A0 A73 L111 | L118 A79 A0 | A0 A79 L118 | A0 A109 | L153 A109 A0 | A0 A115 | L160 A115 A0
sketch "Sketch3" plane through (0, 0, 12) normal (0, 0, 1) x (1, 0, 0)
  circle A0 centre (0, 0) radius 107.5
  circle A1 centre (0, 107.5) radius 2.15
  circle A2 centre (-76.014, 76.014) radius 2.15
  circle A3 centre (-107.5, 0) radius 2.15
  circle A4 centre (-76.014, -76.014) radius 2.15
  circle A5 centre (0, -107.5) radius 2.15
  circle A6 centre (76.014, -76.014) radius 2.15
  circle A7 centre (107.5, 0) radius 2.15
  circle A8 centre (76.014, 76.014) radius 2.15
  dimension "d148" = 215
  dimension "d149" = 4.3
  dimension "d152" = 360
  constraints: 8 centre point, 1 coincident, 1 vertical alignment, 19 other
  measures "d149" diameter of A1
extrude "Extrusion6" cut sketch "Sketch3" against normal through all contours A0 A7 | A0 A7 | A8 A0 | A0 A8 | A6 A0 | A0 A6 | A1 A0 | A0 A1 | A5 A0 | A0 A5 | A2 A0 | A0 A2 | A4 A0 | A0 A4 | A3 A0 | A0 A3
sketch "Sketch4" plane through (0, 0, 14) normal (0, 0, 1) x (1, 0, 0)
  circle A0 centre (0, 0) radius 63.75
  line L0 (0, 0) -> (28.9419, 56.8017)
  line L1 (0, 168) -> (0, -168) projected
  circle A1 centre (28.9419, 56.8017) radius 2.1
  circle A2 centre (-45.0781, 45.0781) radius 2.1
  circle A3 centre (-56.8017, -28.9419) radius 2.1
  circle A4 centre (9.9727, -62.9651) radius 2.1
  circle A5 centre (62.9651, -9.9727) radius 2.1
  circle A6 centre (0, 0) radius 87.5
  line L2 (0, 0) -> (77.9631, 39.7242)
  circle A7 centre (77.9631, 39.7242) radius 2.1
  circle A8 centre (-13.688, 86.4227) radius 2.1
  circle A9 centre (-86.4227, 13.688) radius 2.1
  circle A10 centre (-39.7242, -77.9631) radius 2.1
  circle A11 centre (61.8718, -61.8718) radius 2.1
  dimension "d156" = 127.5
  dimension "d163" = 175
  dimension "d157" = 27
  dimension "d158" = 4.2
  dimension "d161" = 360
  dimension "d164" = 63
  dimension "d165" = 4.2
  dimension "d168" = 360
  constraints: 10 centre point, 4 coincident, 4 end point, 1 point on line, 28 other
  measures "d157" angle of L1 L0
  measures "d158" diameter of A1
  measures "d164" angle of L1 L2
  measures "d165" diameter of A7
extrude "Extrusion7" cut sketch "Sketch4" against normal blind 8 contours A5 A0 | A0 A5 | A1 L0 A0 | A0 A1 | A7 A6 L2 | L2 A6 A7 | L0 A1 A0 | A6 A7 | A4 A0 | A0 A4 | A2 A0 | A0 A2 | A3 A0 | A0 A3 | A8 A6 | A6 A8 | A10 A6 | A6 A10 | A11 A6 | A6 A11 | A9 A6 | A6 A9
sketch "Sketch6" plane through (0, 0, 12) normal (0, 0, 1) x (1, 0, 0)
  line L0 (0, 168) -> (0, -168) projected
  line L1 (69.5236, 89.2106) -> (69.1253, 88.631)
  line L2 (71.3254, 84.4568) -> (66.4388, 77.6061)
  line L3 (9.2853, 110.1546) -> (7.8959, 101.8516)
  line L4 (13.9208, 112.2421) -> (13.7927, 111.5505)
  arc A0 (11.4618, 111.8141) -> (9.2853, 110.1546) centre (11.2579, 109.8245) ccw
  arc A1 (63.5351, 77.2224) -> (9.6749, 99.5309) centre (0, 0) ccw
  arc A2 (69.0767, 91.9424) -> (16.1685, 113.8577) centre (0, 0) ccw
  arc A3 (13.7927, 111.5505) -> (11.4618, 111.8141) centre (0, 0) ccw
  arc A4 (70.9598, 87.1692) -> (69.1253, 88.631) centre (0, 0) ccw
  arc A5 (16.1685, 113.8577) -> (13.9208, 112.2421) centre (15.8873, 111.8776) ccw
  arc A6 (7.8959, 101.8516) -> (9.6749, 99.5309) centre (9.8684, 101.5215) ccw
  arc A7 (63.5351, 77.2224) -> (66.4388, 77.6061) centre (64.8079, 78.7694) ccw
  arc A8 (71.3254, 84.4568) -> (70.9598, 87.1692) centre (69.6971, 85.6182) ccw
  arc A9 (69.5236, 89.2106) -> (69.0767, 91.9424) centre (67.8754, 90.3434) ccw
  line L5 (0, 0) -> (41.1385, 99.317)
  arc A10 (71.651, 84.2245) -> (71.2123, 87.4794) centre (69.6971, 85.6182) ccw
  line L6 (71.651, 84.2245) -> (66.7645, 77.3738)
  arc A11 (63.2809, 76.9135) -> (66.7645, 77.3738) centre (64.8079, 78.7694) ccw
  arc A12 (63.2809, 76.9135) -> (9.6362, 99.1328) centre (0, 0) ccw
  arc A13 (7.5013, 101.9176) -> (9.6362, 99.1328) centre (9.8684, 101.5215) ccw
  line L7 (7.5013, 101.9176) -> (8.8908, 110.2206)
  arc A14 (11.5026, 112.212) -> (8.8908, 110.2206) centre (11.2579, 109.8245) ccw
  arc A15 (13.4679, 111.9931) -> (11.5026, 112.212) centre (0, 0) ccw
  line L8 (13.4679, 111.9931) -> (13.5275, 112.3149)
  arc A16 (16.2248, 114.2537) -> (13.5275, 112.3149) centre (15.8873, 111.8776) ccw
  arc A17 (69.317, 92.2622) -> (16.2248, 114.2537) centre (0, 0) ccw
  arc A18 (69.8533, 88.9841) -> (69.317, 92.2622) centre (67.8754, 90.3434) ccw
  line L9 (69.8533, 88.9841) -> (69.6679, 88.7143)
  arc A19 (71.2123, 87.4794) -> (69.6679, 88.7143) centre (0, 0) ccw
  point P0 (70.9598, 87.1692)
  dimension "d174" = 22.5
  constraints: 1 other
extrude "Extrusion9" cut sketch "Sketch6" against normal through all contours L1 A4 A8 L2 A7 A1 A6 L3 A0 A3 L4 A5 A2 A9 | L6 A11 A12 A13 L7 A14 A15 L8 A16 A17 A18 L9 A19 A10
pattern_circular "Circular Pattern2" count 8 over 360 about axis through (0, 0, -10) along (0, 0, 1) of "Extrusion9"
sketch "Block2" plane through (0, 0, 0) normal (0, 0, 1) x (1, 0, 0)
  line L0 (83.1381, 5.88) -> (71.258, 5.88)
  line L1 (71.258, 5.88) -> (71.258, -6)
  line L2 (71.258, -6) -> (83.1381, -6)
  line L3 (83.1381, -6) -> (83.1381, 5.88)
  line L4 (83.1381, 5.88) -> (71.258, -6) construction
  line L5 (71.258, 5.88) -> (83.1381, -6) construction
  circle A0 centre (77.198, -0.06) radius 2
  circle A1 centre (72.671, -4.587) radius 2.1
  circle A2 centre (81.725, -4.587) radius 2.1
  circle A3 centre (81.725, 4.467) radius 2.1
  circle A4 centre (72.671, 4.467) radius 2.1
  circle A5 centre (70.898, -0.06) radius 0.75
  line L6 (70.898, -0.06) -> (77.198, -0.06)
  dimension "d13" = 11.88
  dimension "d15" = 4.2
  dimension "d12" = 11.88
  dimension "d14" = 4
  dimension "d16" = 1.413
  dimension "d17" = 360
  dimension "d18" = 1.5
  dimension "d19" = 6.3
  constraints: 6 end point, 2 centre point, 2 coincident, 2 midpoint, 1 horizontal, 1 point on line, 21 other
  measures "d12" distance of L5.end L4.end
  measures "d14" diameter of A0
  measures "d18" diameter of A5
  measures "d19" distance of L6.end L6.start
body "Solid1"
